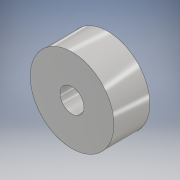
# Autodesk Inventor part: BEARING
Saved by Autodesk Inventor 2017 (Build 210142000, 142)
## iProperties
Created: 2017-09-24
Part Number: BEARING
Material: Generic
Document SubType Name: Modeling
Designer: Alexander Miller
Density: 1 g/cm^3
Appearance: Default
BEARING_A: 7,000 mm
BEARING_B: 2,000 mm
BEARING_C: 3,000 mm
Author: Alexander Miller
Autodesk Inventor part; units mm, degrees
ref_plane "YZ Plane" through (0, 0, 0) normal (1, 0, 0) x (0, 1, 0)
ref_plane "XZ Plane" through (0, 0, 0) normal (0, 1, 0) x (-1, 0, 0)
ref_plane "XY Plane" through (0, 0, 0) normal (0, 0, 1) x (1, 0, 0)
sketch "Sketch1" plane through (0, 0, 0) normal (0, 1, 0) x (-1, 0, 0)
  circle A0 centre (0, 0) radius 3.5
  circle A1 centre (0, 0) radius 1
  dimension "d0" = 2
  dimension "d1" = 7
  constraints: 2 centre point, 1 coincident, 1 concentric
  measures "d0" diameter of A1
  measures "d1" diameter of A0
extrude "Extrusion1" add sketch "Sketch1" along normal blind 3
equation "\"d0\" = BEARING_B"
equation "\"d1\" = BEARING_A"
equation "\"d2\" = BEARING_C"
equation "\"BEARING_A\" = 7"
equation "\"BEARING_B\" = 2"
equation "\"BEARING_C\" = 3"
body "Solid1"
